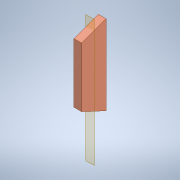
# Autodesk Inventor part: 2x6SupportBracket
Saved by Autodesk Inventor 2022.2 (Build 262287000, 287)
## iProperties
Created: 2021-11-26
Part Number: 2x6SupportBracket
Material: Wood (Walnut)
Document SubType Name: Modeling
Designer: robst
Density: 0.55 g/cm^3
Appearance: Walnut - Natural Polished
Author: robst
Autodesk Inventor part; units mm, degrees
ref_plane "YZ Plane" through (0, 0, 0) normal (1, 0, 0) x (0, 1, 0)
ref_plane "XZ Plane" through (0, 0, 0) normal (0, 1, 0) x (-1, 0, 0)
sketch "Sketch4" plane through (0, 0, 0) normal (1, 0, 0) x (0, 1, 0)
  line L0 (0, 0) -> (-341.2102, 0)
  line L1 (-341.2102, 0) -> (-246.4184, 0)
  line L2 (-406.3534, -139.7) -> (-50.8466, -139.7)
  line L3 (0, 0) -> (50.8466, -139.7)
  line L4 (50.8466, -139.7) -> (-50.8466, -139.7)
  line L5 (-406.3534, -139.7) -> (-341.2102, 0)
  dimension "d17" = 110
  dimension "d19" = 65
  dimension "d20" = 139.7
  dimension "d21" = 457.2
  constraints: 12 end point, 3 horizontal, 1 point on line
  measures "d17" angle of L3 L0
  measures "d19" angle of L2 L5
  measures "d20" distance between parallel lines of L0 L2
  measures "d21" distance of L2.start L3.end
extrude "Extrusion3" add sketch "Sketch4" along normal mid plane 44.45
ref_plane "Work Plane2" through (0, 0, -69.85) normal (0, 0, 1) x (1, 0, 0)
equation "\"d20\" = depth"
equation "\"d21\" = length"
equation "\"d15\" = width"
equation "\"width\" = 44.45"
equation "\"depth\" = 139.7"
equation "\"d18\" = -0.5 * depth"
equation "\"topAngle\" = 20deg"
equation "\"bottomAngle\" = 25deg"
equation "\"length\" = 457.2"
body "Solid2"
